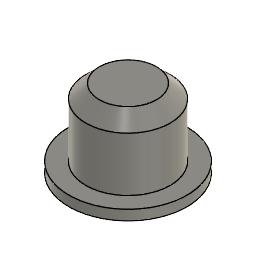
stabilisator_behuizing (Assembly) (Autodesk Fusion 360 archive; units mm, degrees)
design "stabilisator_behuizing_knopje"
Autodesk Fusion 360 part; units mm, degrees
sketch "Sketch1" plane through (0, 0, 0) normal (0, 0, 1) x (1, 0, 0)
  circle A0 centre (0, 0) radius 1.75
  dimension "d1" = 3.5
  constraint coincident A0.centre origin
  measures "d1" diameter of A0
extrude "Extrude1" add sketch "Sketch1" along normal blind 0.3
sketch "Sketch2" plane through (0, 0, 0.3) normal (0, 0, 1) x (-1, 0, 0)
  circle A0 centre (0, 0) radius 1.75
  circle A1 centre (0, 0) radius 1.25
  dimension "d4" = 2.5
  constraint concentric A0 A1
  measures "d4" diameter of A1
extrude "Extrude2" add sketch "Sketch2" along normal blind 2 contours A1
chamfer "Chamfer1" distance 0.4 angle 45 1 edges at (1.1654, 0.452, 2.3)

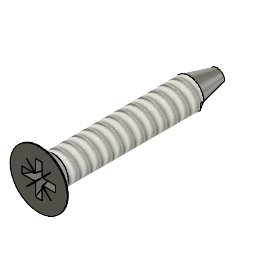
design "Drilling Screw DIN EN ISO 15482 - 2.2 x 13 - Z Steel 4.6 Plain"
description: Drilling Screw DIN EN ISO 15482 - 2.2 x 13 - Z
part number: DIN EN ISO 15482 - 2.2 x 13 - Z Steel 4.6 Plain
Autodesk Fusion 360 part; units mm, degrees
sketch "Sketch1" plane through (0, 0, 0) normal (0, 1, 0) x (1, 0, 0)
  line L0 (0, -2.1522) -> (-2.0862, -2.1522)
  line L1 (-2.0862, -2.1522) -> (-2.0862, -2.0862)
  line L2 (-2.0862, -2.0862) -> (-1.1, -1.1)
  line L3 (-1.1, -1.1) -> (-1.1, 10.8478)
  line L4 (-1.1, 10.8478) -> (0, 10.8478)
  line L5 (0, 10.8478) -> (0, -2.1522)
  dimension "d9" = 2.2
  dimension "d11" = 4.1724
  dimension "d117" = 13
  dimension "d126" = 45
  dimension "d140" = 0.066
  constraint perpendicular L0 L1
  constraint vertical L3
  constraint perpendicular L3 L4
  constraint perpendicular L0 L5
  constraint collinear origin L0.start L4.end
  constraint coincident origin L2
  measures "d117" distance of L0 L4
  measures "d126" angle of L2 L5
  measures "d140" distance of L0 L1.end
revolve "Revolve1" add sketch "Sketch1" angle 360 about axis through (0, 0, -10.8478) along (0, 0, 1) makes body 1
sketch "Sketch7" plane through (0, 0, 2.1522) normal (0, 0, 1) x (1, 0, 0)
  circle A0 centre (0, 0) radius 2.0862
  line L0 (0.2913, 0.2913) -> (0.2913, -0.2913)
  line L1 (-0.2913, 0.2913) -> (0.2913, 0.2913)
  line L2 (-0.2913, -0.2913) -> (-0.2913, 0.2913)
  line L3 (0.2913, -0.2913) -> (-0.2913, -0.2913)
  dimension "d128" = 360
  dimension "d129" = 0.5826
  constraint vertical L0
  constraint coincident L0.start L1.end
  measures "d129" distance of L1 L3
extrude "Extrude4" cut sketch "Sketch7" against normal blind 1.0924 draft -10 contours L0 L1 L2 L3 bodies 1
sketch "Sketch2" plane through (0, 0, 2.1522) normal (0, 0, 1) x (1, 0, 0)
  line L0 (-0.2428, 0.2428) -> (-1.2138, 0.2428)
  line L1 (-1.2138, 0.2428) -> (-1.2138, -0.2428)
  line L2 (-1.2138, -0.2428) -> (-0.2428, -0.2428)
  line L3 (-0.2428, -0.2428) -> (-0.2428, -1.2138)
  line L4 (-0.2428, -1.2138) -> (0.2428, -1.2138)
  line L5 (0.2428, -1.2138) -> (0.2428, -0.2428)
  line L6 (0.2428, -0.2428) -> (1.2138, -0.2428)
  line L7 (1.2138, -0.2428) -> (1.2138, 0.2428)
  line L8 (1.2138, 0.2428) -> (0.2428, 0.2428)
  line L9 (0.2428, 0.2428) -> (0.2428, 1.2138)
  line L10 (0.2428, 1.2138) -> (-0.2428, 1.2138)
  line L11 (-0.2428, 1.2138) -> (-0.2428, 0.2428)
  dimension "d115" = 360
  dimension "d121" = 2.4276
  dimension "d130" = 0.4855
  constraint perpendicular L0 L1
  constraint vertical L0.start L2.end
  constraint horizontal L2
  constraint coincident L0.start L11.end
  measures "d121" distance of L3.end L10
  measures "d130" distance of L0 L2
extrude "Extrude1" add sketch "Sketch2" against normal blind 1.2138 draft -4 separate body makes body 2
draft "Draft1" angle -30 neutral plane through (0, 0, 2.1522) pull (0, 0, 1) 4 faces at (1.1855, 0.0526, 1.7476) (-0.0526, 1.1855, 1.7476) (-0.0526, -1.1855, 1.7476) (-1.1855, -0.0526, 1.7476) on bodies 2
combine "Combine1" operation cut target body 1 tool bodies 2
sketch "Sketch6" plane through (0, 0, 2.1522) normal (0, 0, 1) x (1, 0, 0)
  circle A0 centre (0, 0) radius 2.0862
  line L0 (1.75, 0) -> (22.5, 0) construction
  circle A1 centre (0, 0) radius 1.2378 construction
  line L1 (-0.2913, 0.2913) -> (-0.8753, 0.8753) construction
  line L2 (-0.2428, 0.2913) -> (-0.8753, 0.8753)
  line L3 (-0.2913, 0.2428) -> (-0.8753, 0.8753)
  line L4 (-0.2913, 0.2428) -> (-0.2428, 0.2913)
  line L5 (-0.2913, 0.2428) -> (-0.2913, 0.2913) construction
  line L6 (-0.2913, 0.2913) -> (-0.2428, 0.2913) construction
  point P0 (-0.2428, 1.2138)
  point P1 (-0.2913, 0.2913)
  point P2 (-0.2428, 0.2913)
  point P3 (-0.2913, 0.2428)
  dimension "d100" = 135
  constraint concentric A0 A1
  constraint coincident A1 L1.end
  constraint coincident P2 L2.start
  constraint coincident P3 L3.start
  constraint coincident A1 P0
  constraint coincident P1 L1.start
  measures "d100" angle of L0 L1
extrude "Extrude2" cut sketch "Sketch6" against normal blind 1.2897 draft -30 contours L2 L3 L4 bodies 1
pattern_circular "C-Pattern1" count 4 over 360 about axis through (0, 0, 1.75) along (0, 0, 1) of "Extrude2"
thread "Thread1" "Metric Forming Screw Threads 2.2 2.2x0.8 2.2x0.8 6g" major diameter 2.17 minor diameter 1.575 pitch 0.8 angle 60 resizes the face on face at (-1.0986, 0.0548, -2.8826) on bodies 1
sketch "Sketch5" plane through (0, 0, 0) normal (0, 1, 0) x (1, 0, 0)
  line L0 (-1.122, 10.8478) -> (-1.122, 8.6478)
  line L1 (-1.122, 8.6478) -> (-0.55, 10.8478)
  line L2 (0, 10.8478) -> (0, -2.1522)
  line L3 (-1.122, 10.8478) -> (0, 10.8478)
  dimension "d93" = 1.122
  dimension "d122" = 0.55
  dimension "d123" = 2.2
  constraint vertical L0
  constraint coincident L2.start L3.end
  constraint perpendicular L0 L3
  constraint coincident L1.end L3
  measures "d93" distance of origin L0
  measures "d122" distance of L1.end L2
  measures "d123" distance of L0.end L3
revolve "Revolve2" cut sketch "Sketch5" angle 360 about axis through (0, 0, -10.8478) along (0, 0, 1) bodies 1
sketch "Sketch8" plane through (0, 0, 0) normal (0, 1, 0) x (-1, 0, 0)
  line L0 (0, -10.8478) -> (-1.122, -10.8478)
  line L1 (-1.122, -10.8478) -> (-1.122, -8.5378)
  arc A0 (0, -10.8478) -> (-1.122, -8.5378) centre (-2.9389, -10.8478) ccw
  point P0 (0, -10.8478)
  dimension "d124" = 2.31
  dimension "d125" = 1.122
  constraint perpendicular L0 L1
  constraint coincident L0 A0.centre
  constraint coincident P0 L0.start
  constraint vertical L1
  measures "d124" distance of L0 L1.end
  measures "d125" distance of P0 L1
extrude "Extrude5" cut sketch "Sketch8" against normal blind 1.1 bodies 1
equation "d9 = adsk_nomdia"
equation "d11 = adsk_headdia"
equation "adsk_headang = 90.00 deg"
equation "d31 = -adsk_phildepth"
equation "d61 = -adsk_headh"
equation "d68 = -adsk_phildepth * 0.9"
equation "d83 = -adsk_nomdia / 2"
equation "d93 = adsk_nomdia * 0.51"
equation "d98 = ( adsk_nomdia * 0.5 ) * tan(90 deg - adsk_headang * 0.5) + adsk_headh"
equation "d117 = adsk_nomlen"
equation "d121 = adsk_phildia"
equation "d122 = adsk_endpointdia / 2"
equation "d123 = adsk_startlen"
equation "d124 = adsk_startlen * 1.05"
equation "d125 = adsk_nomdia * 0.51"
equation "d126 = adsk_headang * 0.5"
equation "d129 = adsk_philwidth * 1.2"
equation "d130 = adsk_philwidth"
equation "adsk_nomlen = 13.00 mm"
equation "adsk_headh = 1.2896552 mm"
equation "adsk_headdia = 4.1724138 mm"
equation "adsk_nomdia = 2.20 mm"
equation "adsk_phildia = 2.4275862 mm"
equation "adsk_philwidth = 0.4855172 mm"
equation "adsk_phildepth = 1.2137931 mm"
equation "adsk_startlen = adsk_nomdia"
equation "adsk_endpointdia = adsk_nomdia / 2"
equation "d140 = 0.03 * adsk_nomdia"

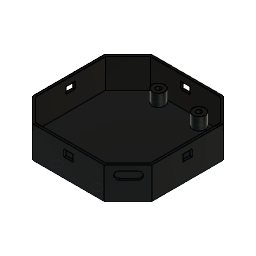
design "stabilisator_behuizing_onderkant"
Autodesk Fusion 360 part; units mm, degrees
sketch "Sketch1" plane through (0, 0, 0) normal (0, 0, 1) x (1, 0, 0)
  line L0 (-26.5, 26.5) -> (26.5, 26.5)
  line L1 (26.5, 26.5) -> (26.5, -26.5)
  line L2 (26.5, -26.5) -> (-26.5, -26.5)
  line L3 (-26.5, -26.5) -> (-26.5, 26.5)
  line L4 (-26.5, 26.5) -> (26.5, -26.5) construction
  line L5 (26.5, 26.5) -> (-26.5, -26.5) construction
  line L6 (-15.8934, 26.5) -> (-26.5, 15.8934)
  line L7 (15.8934, 26.5) -> (26.5, 15.8934)
  line L8 (26.5, -15.8934) -> (15.8934, -26.5)
  line L9 (-26.5, -15.8934) -> (-15.8934, -26.5)
  dimension "d34" = 53
  dimension "d35" = 53
  dimension "d36" = 15
  dimension "d37" = 15
  dimension "d38" = 15
  dimension "d39" = 15
  constraint horizontal L0
  constraint perpendicular L0 L1
  constraint parallel L0 L2
  constraint parallel L1 L3
  constraint coincident L4 origin
  constraint coincident L5 origin
  constraint coincident L0 L6.start
  constraint coincident L3 L6.end
  constraint perpendicular L4 L6
  constraint coincident L0 L7.start
  constraint coincident L1 L7.end
  constraint perpendicular L5 L7
  constraint coincident L1 L8.start
  constraint coincident L2 L8.end
  constraint perpendicular L4 L8
  constraint coincident L3 L9.start
  constraint coincident L2 L9.end
  constraint perpendicular L5 L9
  measures "d34" distance of L0.start L0.end
  measures "d35" distance of L0.start L2.end
  measures "d36" distance of L6.start L6.end
  measures "d37" distance of L7.start L7.end
  measures "d38" distance of L8.start L8.end
  measures "d39" distance of L9.start L9.end
extrude "Extrude1" add sketch "Sketch1" along normal blind 1 contours L0 L1 L2 L3 L6 L7 L8 L9
sketch "Sketch3" plane through (0, 0, 1) normal (0, 0, 1) x (-1, 0, 0)
  line L0 (15.8934, -26.5) -> (26.5, -15.8934)
  line L1 (26.5, -15.8934) -> (26.5, 15.8934)
  line L2 (26.5, 15.8934) -> (15.8934, 26.5)
  line L3 (15.8934, 26.5) -> (-15.8934, 26.5)
  line L4 (-15.8934, 26.5) -> (-26.5, 15.8934)
  line L5 (-26.5, 15.8934) -> (-26.5, -15.8934)
  line L6 (-26.5, -15.8934) -> (-15.8934, -26.5)
  line L7 (-15.8934, -26.5) -> (15.8934, -26.5)
  line L8 (25.5, -25.5) -> (-25.5, -25.5)
  line L9 (-25.5, -25.5) -> (-25.5, 25.5)
  line L10 (-25.5, 25.5) -> (25.5, 25.5)
  line L11 (25.5, 25.5) -> (25.5, -25.5)
  line L12 (25.5, -25.5) -> (-25.5, 25.5) construction
  line L13 (-25.5, -25.5) -> (25.5, 25.5) construction
  line L14 (15.4792, -25.5) -> (25.5, -15.4792)
  line L15 (-15.4792, -25.5) -> (-25.5, -15.4792)
  line L16 (-25.5, 15.4792) -> (-15.4792, 25.5)
  line L17 (15.4792, 25.5) -> (25.5, 15.4792)
  dimension "d42" = 1
  dimension "d43" = 1
  dimension "d44" = 1
  dimension "d45" = 1
  dimension "d46" = 1
  constraint horizontal L8
  constraint perpendicular L8 L9
  constraint parallel L8 L10
  constraint parallel L9 L11
  constraint coincident L12 origin
  constraint coincident L13 origin
  constraint coincident L8 L14.start
  constraint coincident L11 L14.end
  constraint parallel L0 L14
  constraint coincident L8 L15.start
  constraint coincident L9 L15.end
  constraint perpendicular L14 L15
  constraint coincident L9 L16.start
  constraint coincident L10 L16.end
  constraint perpendicular L12 L16
  constraint coincident L10 L17.start
  constraint coincident L11 L17.end
  constraint perpendicular L16 L17
  measures "d42" distance of L0 L14
  measures "d43" distance of L6 L15
  measures "d44" distance of L3 L10
  measures "d45" distance of L4 L16
  measures "d46" distance of L2 L17
extrude "Extrude3" add sketch "Sketch3" along normal blind 13 contours L0 L6 L7 L8 | L0 L8 L11 L14 | L0 L1 L2 L11 | L6 L8 L9 L15 | L4 L5 L6 L9 | L2 L10 L11 L17 | L2 L3 L4 L10 | L4 L9 L10 L16
sketch "Sketch5" plane through (21.1967, -21.1967, 0) normal (0.707107, -0.707107, 0) x (0.707107, 0.707107, 0)
  line L0 (-7.5, 0) -> (7.5, 0)
  line L1 (7.5, 0) -> (7.5, 14)
  line L2 (7.5, 14) -> (-7.5, 14)
  line L3 (-7.5, 14) -> (-7.5, 0)
  line L4 (-2.746, 8.1279) -> (3.1066, 8.15)
  arc A0 (3.1066, 8.15) -> (3.0934, 11.65) centre (3.1, 9.9) ccw
  line L5 (3.0934, 11.65) -> (-2.7592, 11.6279)
  arc A1 (-2.7592, 11.6279) -> (-2.746, 8.1279) centre (-2.7526, 9.8779) ccw
  line L6 (-2.7526, 9.8779) -> (3.1, 9.9) construction
  dimension "d93" = 4.1221
  dimension "d94" = 4.7474
  dimension "d95" = 1.75
  dimension "d96" = 5.8526
  constraint tangent L4 A0
  constraint tangent A0 L5
  constraint parallel L4 L5
  constraint tangent L5 A1
  constraint tangent L4 A1
  measures "d93" distance of L2 A1.centre
  measures "d94" distance of L3 A1.centre
  measures "d95" distance of A1.centre L4
  measures "d96" horizontal distance of A1.centre A0.centre
extrude "Extrude5" cut sketch "Sketch5" against normal blind 2 contours L4 A0 L5 A1
sketch "Sketch7" plane through (0, 26.5, 0) normal (0, 1, 0) x (-1, 0, 0)
  line L0 (-15.8934, 0) -> (15.8934, 0)
  line L1 (15.8934, 0) -> (15.8934, 14)
  line L2 (15.8934, 14) -> (-15.8934, 14)
  line L3 (-15.8934, 14) -> (-15.8934, 0)
  line L4 (-2.0165, 11.171) -> (2.0293, 11.171)
  line L5 (2.0293, 11.171) -> (2.0293, 8.1421)
  line L6 (2.0293, 8.1421) -> (-2.0165, 8.1421)
  line L7 (-2.0165, 8.1421) -> (-2.0165, 11.171)
  dimension "d82" = 2.829
  dimension "d83" = 4.0458
  dimension "d84" = 3.0289
  dimension "d85" = 13.8769
  constraint horizontal L4
  constraint vertical L5
  constraint horizontal L6
  constraint vertical L7
  measures "d82" distance of L2 L4
  measures "d83" distance of L5 L7
  measures "d84" distance of L4 L6
  measures "d85" distance of L3 L7
extrude "Extrude7" cut sketch "Sketch7" against normal through all contours L4 L5 L6 L7
sketch "Sketch8" plane through (-26.5, 0, 0) normal (-1, 0, 0) x (0, -1, 0)
  line L0 (-15.8934, 0) -> (15.8934, 0)
  line L1 (15.8934, 0) -> (15.8934, 14)
  line L2 (15.8934, 14) -> (-15.8934, 14)
  line L3 (-15.8934, 14) -> (-15.8934, 0)
  line L4 (-2.0152, 11.1757) -> (2.0191, 11.1757)
  line L5 (2.0191, 11.1757) -> (2.0191, 8.2313)
  line L6 (2.0191, 8.2313) -> (-2.0152, 8.2313)
  line L7 (-2.0152, 8.2313) -> (-2.0152, 11.1757)
  dimension "d87" = 2.8243
  dimension "d88" = 2.9444
  dimension "d89" = 4.0342
  dimension "d90" = 13.8782
  constraint horizontal L4
  constraint vertical L5
  constraint horizontal L6
  constraint vertical L7
  measures "d87" distance of L2 L4
  measures "d88" distance of L4.start L6.end
  measures "d89" distance of L5.end L6.end
  measures "d90" distance of L3 L7
extrude "Extrude8" cut sketch "Sketch8" against normal through all contours L4 L5 L6 L7
sketch "Sketch9" plane through (0, 0, 1) normal (0, 0, 1) x (-1, 0, 0)
  line L0 (25.5, -15.4792) -> (25.5, 15.4792)
  line L1 (25.5, 15.4792) -> (15.4792, 25.5)
  line L2 (15.4792, 25.5) -> (-15.4792, 25.5)
  line L3 (-15.4792, 25.5) -> (-25.5, 15.4792)
  line L4 (-25.5, 15.4792) -> (-25.5, -15.4792)
  line L5 (-25.5, -15.4792) -> (-15.4792, -25.5)
  line L6 (-15.4792, -25.5) -> (15.4792, -25.5)
  line L7 (15.4792, -25.5) -> (25.5, -15.4792)
  circle A0 centre (-9.009, 22.5618) radius 1.1
  circle A1 centre (9.0089, 22.5618) radius 1.1
  circle A2 centre (-9.009, -22.5547) radius 1.1
  circle A3 centre (9.0089, -22.5547) radius 1.1
  dimension "d62" = 2.2
  dimension "d63" = 2.2
  dimension "d64" = 2.2
  dimension "d65" = 2.2
  measures "d62" diameter of A0
  measures "d63" diameter of A1
  measures "d64" diameter of A2
  measures "d65" diameter of A3
extrude "Extrude9" cut sketch "Sketch9" against normal blind 10 contours A0 | A1 | A2 | A3
chamfer "Chamfer1" distance 1 angle 45 4 edges at (-7.9834, 22.9525, 0) (10.0345, 22.9525, 0) (10.0345, -22.164, 0) (-7.9834, -22.164, 0)
sketch "Sketch11" plane through (-21.1967, -21.1967, 0) normal (-0.707107, -0.707107, 0) x (0.707107, -0.707107, 0)
  line L0 (-7.5, 0) -> (7.5, 0)
  line L1 (7.5, 0) -> (7.5, 14)
  line L2 (7.5, 14) -> (-7.5, 14)
  line L3 (-7.5, 14) -> (-7.5, 0)
  circle A0 centre (0.0835, 9.893) radius 1.5
  dimension "d73" = 3
  dimension "d91" = 4.107
  dimension "d92" = 7.5835
  measures "d73" diameter of A0
  measures "d91" distance of L2 A0.centre
  measures "d92" distance of L3 A0.centre
extrude "Extrude11" cut sketch "Sketch11" against normal blind 5 contours A0
sketch "Sketch12" plane through (-20.4896, -20.4896, 0) normal (0.707107, 0.707107, 0) x (-0.707107, 0.707107, 0)
  circle A0 centre (-0.0835, 9.893) radius 1.5
  line L0 (-7.0858, 1) -> (7.0858, 1)
  line L1 (7.0858, 1) -> (7.0858, 14)
  line L2 (7.0858, 14) -> (-7.0858, 14)
  line L3 (-7.0858, 14) -> (-7.0858, 1)
  circle A1 centre (-0.0835, 9.893) radius 1.5
  circle A2 centre (-0.0835, 9.893) radius 2
  dimension "d77" = 4
  constraint concentric A0 A1
  constraint concentric A1 A2
  measures "d77" diameter of A2
extrude "Extrude12" cut sketch "Sketch12" against normal blind 0.5 contours A2
sketch "Sketch13" plane through (0, 0, 0) normal (0, 0, -1) x (1, 0, 0)
  circle A0 centre (9.009, 22.5618) radius 2.1
  circle A1 centre (-9.0089, -22.5547) radius 2.1
  line L0 (-26.5, -15.8934) -> (-15.8934, -26.5)
  line L1 (-15.8934, -26.5) -> (15.8934, -26.5)
  line L2 (15.8934, -26.5) -> (26.5, -15.8934)
  line L3 (26.5, -15.8934) -> (26.5, 15.8934)
  line L4 (26.5, 15.8934) -> (15.8934, 26.5)
  line L5 (15.8934, 26.5) -> (-15.8934, 26.5)
  line L6 (-15.8934, 26.5) -> (-26.5, 15.8934)
  line L7 (-26.5, 15.8934) -> (-26.5, -15.8934)
  circle A2 centre (9.009, -22.5547) radius 2.1
  circle A3 centre (-9.0089, 22.5618) radius 2.1
sketch "Sketch14" plane through (0, 0, 1) normal (0, 0, 1) x (-1, 0, 0)
  line L0 (25.5, -15.4792) -> (25.5, 15.4792)
  line L1 (25.5, 15.4792) -> (15.4792, 25.5)
  line L2 (15.4792, 25.5) -> (-15.4792, 25.5)
  line L3 (-15.4792, 25.5) -> (-25.5, 15.4792)
  line L4 (-25.5, 15.4792) -> (-25.5, -15.4792)
  line L5 (-25.5, -15.4792) -> (-15.4792, -25.5)
  line L6 (-15.4792, -25.5) -> (15.4792, -25.5)
  line L7 (15.4792, -25.5) -> (25.5, -15.4792)
  circle A0 centre (9.0089, -22.5547) radius 1.1
  circle A1 centre (9.0089, -22.5547) radius 2.75
  circle A2 centre (-9.009, -22.5547) radius 1.1
  circle A3 centre (-9.009, -22.5547) radius 2.75
  circle A4 centre (9.0089, 22.5618) radius 1.1
  circle A5 centre (9.0089, 22.5618) radius 2.75
  circle A6 centre (-9.009, 22.5618) radius 1.1
  circle A7 centre (-9.009, 22.5618) radius 2.75
  circle A8 centre (9.0089, 22.5618) radius 1.1
  circle A9 centre (9.0089, -22.5547) radius 1.1
  circle A10 centre (-9.009, 22.5618) radius 1.1
  circle A11 centre (-9.009, -22.5547) radius 1.1
  dimension "d97" = 5.5
  dimension "d98" = 5.5
  dimension "d99" = 5.5
  dimension "d100" = 5.5
  constraint concentric A2 A3
  constraint concentric A4 A5
  constraint concentric A6 A7
  measures "d97" diameter of A1
  measures "d98" diameter of A3
  measures "d99" diameter of A5
  measures "d100" diameter of A7
extrude "Extrude13" add sketch "Sketch14" along normal blind 5.5 contours A1 | A3 | A5 | A7
